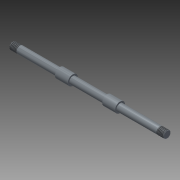
# Autodesk Inventor part: 刮肉轮轴
Saved by Autodesk Inventor 2015 (Build 190159000, 159)
## iProperties
Created: 2017-05-22
Part Number: 刮肉轮轴
Material: 常规
Document SubType Name: Modeling
Designer: Administrator
Density: 1 g/cm^3
Appearance: 锌
Author: Administrator
Autodesk Inventor part; units mm, degrees
ref_plane "YZ Plane" through (0, 0, 0) normal (1, 0, 0) x (0, 1, 0)
ref_plane "XZ Plane" through (0, 0, 0) normal (0, 1, 0) x (-1, 0, 0)
ref_plane "XY Plane" through (0, 0, 0) normal (0, 0, 1) x (1, 0, 0)
sketch "草图1" plane through (0, 0, 0) normal (0, 0, 1) x (1, 0, 0)
  line L0 (0, 0) -> (0, 2.5)
  line L1 (0, 2.5) -> (5, 2.5)
  line L2 (5, 2.5) -> (33, 2.5)
  line L3 (33, 2.5) -> (33, 3.5)
  line L4 (33, 3.5) -> (42, 3.5)
  line L5 (42, 3.5) -> (42, 2.5)
  line L6 (42, 2.5) -> (66, 2.5)
  line L7 (66, 2.5) -> (66, 3.5)
  line L8 (66, 3.5) -> (75, 3.5)
  line L9 (75, 3.5) -> (75, 2.5)
  line L10 (75, 2.5) -> (108, 2.5)
  line L11 (108, 2.5) -> (108, 0)
  line L12 (108, 0) -> (0, 0)
  line L13 (-21.6, 0) -> (129.6, 0) projected
  dimension "d0" = 2.5
  dimension "d1" = 5
  dimension "d2" = 28
  dimension "d3" = 1
  dimension "d4" = 9
  dimension "d5" = 24
  dimension "d6" = 9
  dimension "d7" = 33
  constraints: 26 end point, 8 perpendicular, 7 point on line, 1 vertical
  measures "d0" distance of L0.start L0.end
  measures "d1" distance of L0.end L1.end
  measures "d2" distance of L1.end L2.end
  measures "d3" distance of L2.end L3.end
  measures "d4" distance of L3.end L4.end
  measures "d5" distance of L5.end L6.end
  measures "d6" distance of L7.end L8.end
  measures "d7" distance of L9.end L10.end
revolve "旋转1" add sketch "草图1" angle 360 about axis through (-10, 0, 0) along (1, 0, 0)
thread "螺纹1" size "M5x0.8" class "6g" standard "ANSI Metric M Profile" length 5
thread "螺纹2" size "M5x0.8" class "6g" standard "ANSI Metric M Profile" length 5
chamfer "倒角1" distance 0.25 angle 45 2 edges at (108, -2.5, 0) (0, -2.5, 0)
